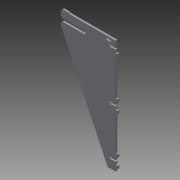
# Autodesk Inventor part: support1_import
Saved by Autodesk Inventor 2015 (Build 190159000, 159)
## iProperties
Created: 2015-04-20
Part Number: support1_import
Material: Generic
Document SubType Name: Modeling
Designer: X
Density: 1 g/cm^3
Appearance: Default
Author: X
Autodesk Inventor part; units mm, degrees
ref_plane "YZ Plane" through (0, 0, 0) normal (1, 0, 0) x (0, 1, 0)
ref_plane "XZ Plane" through (0, 0, 0) normal (0, 1, 0) x (-1, 0, 0)
ref_plane "XY Plane" through (0, 0, 0) normal (0, 0, 1) x (1, 0, 0)
sketch "Sketch1" plane through (0, 0, 0) normal (0, 1, 0) x (-1, 0, 0)
  line L0 (222.5841, 183.0318) -> (224.5841, 185.0318)
  line L1 (224.5841, 185.0318) -> (244.5841, 185.0318)
  line L2 (244.5841, 185.0318) -> (249.5841, 180.0318)
  line L3 (249.5841, 180.0318) -> (249.5841, 164.4318)
  line L4 (249.5841, 164.4318) -> (244.5841, 159.4318)
  line L5 (244.5841, 159.4318) -> (174.5841, 159.4318)
  line L6 (174.5841, 159.4318) -> (173.4453, 159.2819)
  line L7 (173.4453, 159.2819) -> (172.3841, 158.8423)
  line L8 (172.3841, 158.8423) -> (171.4728, 158.1431)
  line L9 (171.4728, 158.1431) -> (170.7736, 157.2318)
  line L10 (170.7736, 157.2318) -> (170.334, 156.1706)
  line L11 (170.334, 156.1706) -> (170.1841, 155.0318)
  line L12 (170.1841, 155.0318) -> (170.334, 153.893)
  line L13 (170.334, 153.893) -> (170.7736, 152.8318)
  line L14 (170.7736, 152.8318) -> (171.4728, 151.9206)
  line L15 (171.4728, 151.9206) -> (172.3841, 151.2213)
  line L16 (172.3841, 151.2213) -> (173.4453, 150.7818)
  line L17 (173.4453, 150.7818) -> (174.5841, 150.6318)
  line L18 (174.5841, 150.6318) -> (244.5841, 150.6318)
  line L19 (244.5841, 150.6318) -> (249.5841, 145.6318)
  line L20 (249.5841, 145.6318) -> (249.5841, 138.0318)
  line L21 (249.5841, 138.0318) -> (97.1841, -184.9681)
  line L22 (97.1841, -184.9681) -> (71.7841, -184.9681)
  line L23 (71.7841, -184.9681) -> (71.7841, -175.6109)
  line L24 (71.7841, -175.6109) -> (65.6841, -175.6109)
  line L25 (65.6841, -175.6109) -> (65.6841, -166.8109)
  line L26 (65.6841, -166.8109) -> (71.7841, -166.8109)
  line L27 (71.7841, -166.8109) -> (71.7841, -157.2531)
  line L28 (71.7841, -157.2531) -> (83.7841, -157.2531)
  line L29 (83.7841, -157.2531) -> (83.7841, -159.0531)
  line L30 (83.7841, -159.0531) -> (88.8841, -159.0531)
  line L31 (88.8841, -159.0531) -> (88.8841, -157.2531)
  line L32 (88.8841, -157.2531) -> (92.8841, -157.2531)
  line L33 (92.8841, -157.2531) -> (92.8841, -152.8531)
  line L34 (92.8841, -152.8531) -> (88.8841, -152.8531)
  line L35 (88.8841, -152.8531) -> (88.8841, -151.0531)
  line L36 (88.8841, -151.0531) -> (83.7841, -151.0531)
  line L37 (83.7841, -151.0531) -> (83.7841, -152.8531)
  line L38 (83.7841, -152.8531) -> (71.7841, -152.8531)
  line L39 (71.7841, -152.8531) -> (71.7841, -143.3109)
  line L40 (71.7841, -143.3109) -> (65.6841, -143.3109)
  line L41 (65.6841, -143.3109) -> (65.6841, -134.5109)
  line L42 (65.6841, -134.5109) -> (71.7841, -134.5109)
  line L43 (71.7841, -134.5109) -> (71.7841, -20.5182)
  line L44 (71.7841, -20.5182) -> (65.6841, -20.5182)
  line L45 (65.6841, -20.5182) -> (65.6841, -11.7182)
  line L46 (65.6841, -11.7182) -> (71.7841, -11.7182)
  line L47 (71.7841, -11.7182) -> (71.7841, -2.1682)
  line L48 (71.7841, -2.1682) -> (83.7841, -2.1682)
  line L49 (83.7841, -2.1682) -> (83.7841, -3.9682)
  line L50 (83.7841, -3.9682) -> (88.8841, -3.9682)
  line L51 (88.8841, -3.9682) -> (88.8841, -2.1682)
  line L52 (88.8841, -2.1682) -> (92.8841, -2.1682)
  line L53 (92.8841, -2.1682) -> (92.8841, 2.2318)
  line L54 (92.8841, 2.2318) -> (88.8841, 2.2318)
  line L55 (88.8841, 2.2318) -> (88.8841, 4.0318)
  line L56 (88.8841, 4.0318) -> (83.7841, 4.0318)
  line L57 (83.7841, 4.0318) -> (83.7841, 2.2318)
  line L58 (83.7841, 2.2318) -> (71.7841, 2.2318)
  line L59 (71.7841, 2.2318) -> (71.7841, 11.7818)
  line L60 (71.7841, 11.7818) -> (65.6841, 11.7818)
  line L61 (65.6841, 11.7818) -> (65.6841, 20.5818)
  line L62 (65.6841, 20.5818) -> (71.7841, 20.5818)
  line L63 (71.7841, 20.5818) -> (71.7841, 139.4819)
  line L64 (71.7841, 139.4819) -> (65.6841, 139.4819)
  line L65 (65.6841, 139.4819) -> (65.6841, 148.2819)
  line L66 (65.6841, 148.2819) -> (71.7841, 148.2819)
  line L67 (71.7841, 148.2819) -> (71.7841, 157.8374)
  line L68 (71.7841, 157.8374) -> (83.7841, 157.8374)
  line L69 (83.7841, 157.8374) -> (83.7841, 156.0374)
  line L70 (83.7841, 156.0374) -> (88.8841, 156.0374)
  line L71 (88.8841, 156.0374) -> (88.8841, 157.8374)
  line L72 (88.8841, 157.8374) -> (92.8841, 157.8374)
  line L73 (92.8841, 157.8374) -> (92.8841, 162.2374)
  line L74 (92.8841, 162.2374) -> (88.8841, 162.2374)
  line L75 (88.8841, 162.2374) -> (88.8841, 164.0374)
  line L76 (88.8841, 164.0374) -> (83.7841, 164.0374)
  line L77 (83.7841, 164.0374) -> (83.7841, 162.2374)
  line L78 (83.7841, 162.2374) -> (71.7841, 162.2374)
  line L79 (71.7841, 162.2374) -> (71.7841, 183.0318)
  line L80 (71.7841, 183.0318) -> (222.5841, 183.0318)
  line L81 (102.5454, 172.2034) -> (101.717, 171.5677)
  line L82 (101.717, 171.5677) -> (100.7523, 171.1681)
  line L83 (100.7523, 171.1681) -> (99.717, 171.0318)
  line L84 (99.717, 171.0318) -> (91.721, 171.0318)
  line L85 (91.721, 171.0318) -> (90.6857, 171.1681)
  line L86 (90.6857, 171.1681) -> (89.721, 171.5677)
  line L87 (89.721, 171.5677) -> (88.8926, 172.2034)
  line L88 (88.8926, 172.2034) -> (88.2569, 173.0318)
  line L89 (88.2569, 173.0318) -> (87.8573, 173.9965)
  line L90 (87.8573, 173.9965) -> (87.721, 175.0318)
  line L91 (87.721, 175.0318) -> (87.8573, 176.0671)
  line L92 (87.8573, 176.0671) -> (88.2569, 177.0318)
  line L93 (88.2569, 177.0318) -> (88.8926, 177.8603)
  line L94 (88.8926, 177.8603) -> (89.721, 178.4959)
  line L95 (89.721, 178.4959) -> (90.6857, 178.8955)
  line L96 (90.6857, 178.8955) -> (91.721, 179.0318)
  line L97 (91.721, 179.0318) -> (99.7838, 179.0318)
  line L98 (99.7838, 179.0318) -> (100.7523, 178.8955)
  line L99 (100.7523, 178.8955) -> (101.717, 178.4959)
  line L100 (101.717, 178.4959) -> (102.5454, 177.8603)
  line L101 (102.5454, 177.8603) -> (103.1811, 177.0318)
  line L102 (103.1811, 177.0318) -> (103.5807, 176.0671)
  line L103 (103.5807, 176.0671) -> (103.717, 175.0318)
  line L104 (103.717, 175.0318) -> (103.5807, 173.9965)
  line L105 (103.5807, 173.9965) -> (103.1811, 173.0318)
  line L106 (103.1811, 173.0318) -> (102.5454, 172.2034)
  constraints: 214 end point
extrude "Extrusion1" add sketch "Sketch1" along normal blind 6
body "Solid1"
